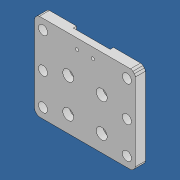
# Autodesk Inventor part: Diode_Laser_Mount
Saved by Autodesk Inventor 2020 (Build 240168000, 168)
## iProperties
Created: 2021-07-14
Part Number: Diode_Laser_Mount
Material: 一般
Document SubType Name: Modeling
Designer: ken113
Density: 1 g/cm^3
Appearance: 既定
Author: ken113
Autodesk Inventor part; units mm, degrees
ref_plane "YZ Plane" through (0, 0, 0) normal (1, 0, 0) x (0, 1, 0)
ref_plane "XZ Plane" through (0, 0, 0) normal (0, 1, 0) x (-1, 0, 0)
ref_plane "XY Plane" through (0, 0, 0) normal (0, 0, 1) x (1, 0, 0)
sketch "スケッチ1" plane through (0, 0, 0) normal (0, 0, 1) x (1, 0, 0)
  line L0 (30, -26) -> (-30, -26)
  line L1 (-30, -26) -> (-30, 26)
  line L2 (-30, 26) -> (30, 26)
  line L3 (30, 26) -> (30, -26)
  line L4 (30, -26) -> (-30, 26) construction
  line L5 (-30, -26) -> (30, 26) construction
  point P0 (0, 0)
  dimension "d0" = 60
  dimension "d1" = 52
  constraints: 12 end point, 2 midpoint, 2 parallel, 1 horizontal, 1 perpendicular
  measures "d0" distance of L1.end L2.end
  measures "d1" distance of L0.end L1.end
extrude "押し出し1" add sketch "スケッチ1" along normal blind 6
sketch "スケッチ2" plane through (0, 0, 6) normal (0, 0, 1) x (1, 0, 0)
  line L0 (25, -20) -> (-25, -20)
  line L1 (-25, -20) -> (-25, 20)
  line L2 (-25, 20) -> (25, 20)
  line L3 (25, 20) -> (25, -20)
  line L4 (25, -20) -> (-25, 20) construction
  line L5 (-25, -20) -> (25, 20) construction
  line L6 (-30, -26) -> (30, -26) projected
  point P0 (0, 0)
  point P1 (0, 0)
  point P2 (-25, -1)
  point P3 (25, -1)
  dimension "d4" = 50
  dimension "d5" = 40
  dimension "d6" = 6
  constraints: 12 end point, 4 coincident, 2 midpoint, 2 parallel, 2 point on line, 1 horizontal, 1 perpendicular
  measures "d4" distance of L0.start L0.end
  measures "d5" distance of L2.end L0.start
  measures "d6" distance between parallel lines of L0 L6
hole "穴1" at (-25, -1, 6) at (25, -1, 6) at (25, 20, 6) at (-25, 20, 6) at (-25, -20, 6) at (25, -20, 6) direction (0, 0, -1) diameter 5.4 depth 8.8
sketch "スケッチ3" plane through (0, 0, 6) normal (0, 0, 1) x (1, 0, 0)
  line L0 (-10, -16) -> (10, -16)
  line L1 (10, -16) -> (10, 4)
  line L2 (10, 4) -> (-10, 4)
  line L3 (-10, 4) -> (-10, -16)
  line L4 (-10, -16) -> (10, 4) construction
  line L5 (10, -16) -> (-10, 4) construction
  line L6 (-30, -26) -> (30, -26) projected
  point P0 (0, 0)
  point P1 (0, -6)
  dimension "d14" = 20
  dimension "d15" = 20
  dimension "d16" = 10
  constraints: 12 end point, 2 midpoint, 2 parallel, 1 horizontal, 1 perpendicular
  measures "d14" distance of L2.end L1.end
  measures "d15" distance of L1.end L0.end
  measures "d16" distance between parallel lines of L0 L6
hole "穴2" at (-10, -16, 6) at (-10, 4, 6) at (10, 4, 6) at (10, -16, 6) direction (0, 0, -1) diameter 3.3 depth 8.8 counterbore diameter 6.5 counterbore depth 4
sketch "スケッチ4" plane through (0, 0, 0) normal (0, 0, -1) x (-1, 0, 0)
  circle A0 centre (-10, 4) radius 1.65 projected
  circle A1 centre (10, -16) radius 1.65 projected
  circle A2 centre (10, 4) radius 1.65 projected
  circle A3 centre (-10, -16) radius 1.65 projected
  circle A4 centre (25, -20) radius 2.7 projected
  circle A5 centre (-25, 20) radius 2.7 projected
  circle A6 centre (25, -1) radius 2.7 projected
  circle A7 centre (-25, -1) radius 2.7 projected
  circle A8 centre (25, 20) radius 2.7 projected
  circle A9 centre (-25, -20) radius 2.7 projected
  line L0 (-30, -26) -> (-30, 26) projected
  line L1 (30, -26) -> (-30, -26) projected
  line L2 (30, 26) -> (30, -26) projected
  line L3 (-30, 26) -> (30, 26) projected
  line L4 (-30, 26) -> (30, 26) projected
  line L5 (-11, 26) -> (11, 26)
  line L6 (11, 26) -> (11, 8)
  line L7 (11, 8) -> (-11, 8)
  line L8 (-11, 8) -> (-11, 26)
  point P0 (0, 0)
  point P1 (11, 26)
  point P2 (-11, 26)
  dimension "d24" = 22
  dimension "d25" = 18
  dimension "d26" = 11
  constraints: 8 end point, 2 parallel, 1 horizontal, 1 perpendicular, 1 point on line
  measures "d24" distance of L6.end L7.end
  measures "d25" distance of L5.end L6.end
  measures "d26" distance from line of point (0, 0) L8
extrude "押し出し2" cut sketch "スケッチ4" against normal blind 2 contours L3 L6 L7 L8
chamfer "面取り1" distance 2 angle 45 4 edges at (-30, 26, 3) (-30, -26, 3) (30, -26, 3) (30, 26, 3)
fillet "フィレット1" radius 2 8 edges at (30, 24, 3) (28, 26, 3) (-28, 26, 3) (-30, 24, 3) (-30, -24, 3) (-28, -26, 3) (28, -26, 3) (30, -24, 3)
sketch "スケッチ5" plane through (0, 0, 2) normal (0, 0, -1) x (-1, 0, 0)
  line L0 (11, 26) -> (11, 8) projected
  line L1 (-11, 26) -> (11, 26) projected
  line L2 (-11, 8) -> (-11, 26) projected
  line L3 (11, 8) -> (-11, 8) projected
  point P0 (0, 0)
  point P1 (-4.75, 20)
  point P2 (4.75, 20)
  dimension "d33" = 9.5
  dimension "d34" = 4.75
  dimension "d35" = 6
  constraints: 1 horizontal alignment
  measures "d33" distance of point (4.75, 20) point (-4.75, 20)
  measures "d34" horizontal distance of point (0, 0) point (-4.75, 20)
  measures "d35" distance from line of L1 point (-4.75, 20)
hole "穴3" at (4.75, 20, 2) at (-4.75, 20, 2) direction (0, 0, 1) diameter 1.9 depth 8.8
fillet "フィレット2" radius 2 2 edges at (11, 8, 1) (-11, 8, 1)
